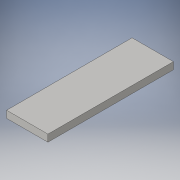
# Autodesk Inventor part: Bread Board
Saved by Autodesk Inventor 2016 (Build 200138000, 138)
## iProperties
Created: 2016-10-07
Part Number: Bread Board
Material: Generic
Document SubType Name: Modeling
Designer: sheehm
Density: 1 g/cm^3
Appearance: Default
Author: sheehm
Autodesk Inventor part; units mm, degrees
ref_plane "YZ Plane" through (0, 0, 0) normal (1, 0, 0) x (0, 1, 0)
ref_plane "XZ Plane" through (0, 0, 0) normal (0, 1, 0) x (-1, 0, 0)
ref_plane "XY Plane" through (0, 0, 0) normal (0, 0, 1) x (1, 0, 0)
sketch "Sketch1" plane through (0, 0, 0) normal (0, 1, 0) x (-1, 0, 0)
  line L0 (6.4246, 18.3268) -> (-48.7954, 18.3268)
  line L1 (-48.7954, 18.3268) -> (-48.7954, 185.9668)
  line L2 (-48.7954, 185.9668) -> (6.4246, 185.9668)
  line L3 (6.4246, 185.9668) -> (6.4246, 18.3268)
  point P0 (0, 0)
  dimension "d0" = 55.22
  dimension "d1" = 167.64
  constraints: 8 end point, 2 parallel, 1 horizontal, 1 perpendicular
  measures "d0" distance of L1.end L2.end
  measures "d1" distance of L0.end L1.end
extrude "Extrusion1" add sketch "Sketch1" along normal blind 9.4
body "Solid1"
